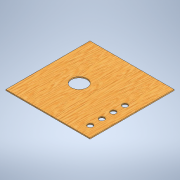
# Autodesk Inventor part: ОСНОВАФАНЕРА
Saved by Autodesk Inventor 2022.4 (Build 264492010, 492A)
## iProperties
Created: 2023-02-19
Part Number: ОСНОВАФАНЕРА
Material: Пиломатериалы — ламинированный шпон
Document SubType Name: Modeling
Designer: artyo
Density: 0.51 g/cm^3
Appearance: Фанера — новая
Author: artyo
Autodesk Inventor part; units mm, degrees
ref_plane "YZ Plane" through (0, 0, 0) normal (1, 0, 0) x (0, 1, 0)
ref_plane "XZ Plane" through (0, 0, 0) normal (0, 1, 0) x (-1, 0, 0)
ref_plane "XY Plane" through (0, 0, 0) normal (0, 0, 1) x (1, 0, 0)
sketch "Эскиз1" plane through (0, 0, 0) normal (0, 1, 0) x (-1, 0, 0)
  line L0 (500, -300) -> (500, 500)
  line L1 (500, 500) -> (-300, 500)
  line L2 (500, -300) -> (-300, -300)
  line L3 (-300, -300) -> (-300, 500)
  point P0 (0, 0)
  point P1 (-300, 300)
  constraints: 8 end point, 1 perpendicular, 1 point on line
extrude "Выдавливание1" add sketch "Эскиз1" along normal blind 10
sketch "Эскиз3" plane through (0, 10, 0) normal (0, 1, 0) x (1, 0, 0)
  circle A0 centre (-203.3931, -99.1972) radius 75
  point P0 (0, 0)
  dimension "d6" = 150
  constraints: 1 centre point
  measures "d6" diameter of A0
extrude "Выдавливание2" cut sketch "Эскиз3" against normal blind 754.25
sketch "Эскиз4" plane through (0, 10, 0) normal (0, 1, 0) x (1, 0, 0)
  circle A0 centre (198.405, -395.8751) radius 25
  circle A1 centre (198.405, -285.8751) radius 25
  circle A2 centre (198.405, -65.8751) radius 25
  circle A3 centre (198.405, -175.8751) radius 25
  point P0 (0, 0)
  dimension "d9" = 50
  dimension "d10" = 50
  dimension "d11" = 50
  dimension "d12" = 50
  dimension "d15" = 110
  dimension "d16" = 110
  dimension "d17" = 110
  constraints: 4 centre point
  measures "d9" diameter of A0
  measures "d10" diameter of A1
  measures "d11" diameter of A2
  measures "d12" diameter of A3
  measures "d15" distance of A0.centre A1.centre
  measures "d16" distance of A3.centre A1.centre
  measures "d17" distance of A3.centre A2.centre
extrude "Выдавливание3" cut sketch "Эскиз4" against normal blind 754.25
